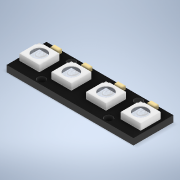
# Autodesk Inventor part: LED WS2812B
Saved by Autodesk Inventor 2020.1 (Build 241239000, 239)
## iProperties
Created: 2019-08-13
Part Number: LED WS2812B
Material: Generic
Document SubType Name: Modeling
Designer: Petar
Density: 1 g/cm^3
Appearance: Default
Author: Petar
Autodesk Inventor part; units mm, degrees
ref_plane "YZ Plane" through (0, 0, 0) normal (1, 0, 0) x (0, 1, 0)
ref_plane "XZ Plane" through (0, 0, 0) normal (0, 1, 0) x (-1, 0, 0)
sketch "Sketch1" plane through (0, 0, 0) normal (0, 1, 0) x (-1, 0, 0)
  line L0 (15.92, 5) -> (-15.92, 5)
  line L1 (-15.92, 5) -> (-15.92, -5)
  line L2 (-15.92, -5) -> (15.92, -5)
  line L3 (15.92, -5) -> (15.92, 5)
  line L4 (15.92, 5) -> (-15.92, -5) construction
  line L5 (-15.92, 5) -> (15.92, -5) construction
  line L6 (-10.87, -4.5) -> (-12.72, -4.5)
  line L7 (-12.72, -4.5) -> (-12.72, -3.5)
  line L8 (-12.72, -3.5) -> (-10.87, -3.5)
  line L9 (-10.87, -3.5) -> (-10.87, -4.5)
  circle A0 centre (-8.42, -3.75) radius 1
  line L10 (15.92, 0) -> (-15.92, 0) construction
  line L11 (0, -5) -> (0, 5) construction
  circle A1 centre (-8.42, 3.75) radius 1
  line L12 (-10.22, -2.5) -> (-15.22, -2.5)
  line L13 (-15.22, -2.5) -> (-15.22, 2.5)
  line L14 (-15.22, 2.5) -> (-10.22, 2.5)
  line L15 (-10.22, 2.5) -> (-10.22, -2.5)
  line L16 (-1.52, -2.5) -> (-6.52, -2.5)
  line L17 (-6.52, -2.5) -> (-6.52, 2.5)
  line L18 (-6.52, 2.5) -> (-1.52, 2.5)
  line L19 (-1.52, 2.5) -> (-1.52, -2.5)
  line L20 (7.18, -2.5) -> (2.18, -2.5)
  line L21 (2.18, -2.5) -> (2.18, 2.5)
  line L22 (2.18, 2.5) -> (7.18, 2.5)
  line L23 (7.18, 2.5) -> (7.18, -2.5)
  line L24 (15.22, -2.5) -> (10.22, -2.5)
  line L25 (10.22, -2.5) -> (10.22, 2.5)
  line L26 (10.22, 2.5) -> (15.22, 2.5)
  line L27 (15.22, 2.5) -> (15.22, -2.5)
  circle A2 centre (8.42, -3.75) radius 1
  circle A3 centre (8.42, 3.75) radius 1
  line L28 (-2.57, -4.5) -> (-4.42, -4.5)
  line L29 (-4.42, -4.5) -> (-4.42, -3.5)
  line L30 (-4.42, -3.5) -> (-2.57, -3.5)
  line L31 (-2.57, -3.5) -> (-2.57, -4.5)
  line L32 (5.73, -4.5) -> (3.88, -4.5)
  line L33 (3.88, -4.5) -> (3.88, -3.5)
  line L34 (3.88, -3.5) -> (5.73, -3.5)
  line L35 (5.73, -3.5) -> (5.73, -4.5)
  line L36 (13.42, -4.5) -> (11.57, -4.5)
  line L37 (11.57, -4.5) -> (11.57, -3.5)
  line L38 (11.57, -3.5) -> (13.42, -3.5)
  line L39 (13.42, -3.5) -> (13.42, -4.5)
  point P0 (0, 0)
  dimension "d0" = 31.84
  dimension "d1" = 10
  dimension "d2" = 1.85
  dimension "d3" = 1
  dimension "d4" = 7.5
  dimension "d5" = 7.5
  dimension "d6" = 2
  dimension "d7" = 3.2
  dimension "d8" = 0.5
  dimension "d9" = 5
  dimension "d10" = 0.7
  dimension "d11" = 3.7
  dimension "d12" = 0.7
  dimension "d14" = 6.45
  dimension "d15" = 6.45
  dimension "d16" = 2.5
  dimension "d18" = 3.7
  constraints: 80 end point, 18 parallel, 13 equal length, 9 horizontal, 9 perpendicular, 6 midpoint, 4 centre point, 3 symmetric about line, 2 collinear, 1 point on line, 7 other
  measures "d0" distance of L2.end L1.end
  measures "d1" distance of L1.end L0.end
  measures "d2" distance of L7.end L8.end
  measures "d3" distance of L6.end L7.end
  measures "d4" distance from line of L1 A0.centre
  measures "d5" distance of A1.centre A0.centre
  measures "d6" diameter of A0
  measures "d7" distance between parallel lines of L7 L1
  measures "d8" distance between parallel lines of L2 L6
  measures "d9" distance between parallel lines of L14 L12
  measures "d10" distance between parallel lines of L1 L13
  measures "d11" distance between parallel lines of L15 L17
  measures "d12" distance between parallel lines of L3 L27
  measures "d14" distance between parallel lines of L9 L29
  measures "d15" distance between parallel lines of L31 L33
  measures "d16" distance between parallel lines of L3 L39
  measures "d18" distance between parallel lines of L19 L21
extrude "Extrusion1" add sketch "Sketch1" against normal blind 1.6 contours L3 L2 L1 L0 | L6 L7 L8 L9 | L12 L13 L14 L15 | L16 L17 L18 L19 | L20 L21 L22 L23 | L24 L25 L26 L27 | L28 L29 L30 L31 | L32 L33 L34 L35 | L36 L37 L38 L39
extrude "Extrusion2" add sketch "Sketch1" along normal blind 1.6 contours L12 L13 L14 L15 | L16 L17 L18 L19 | L20 L21 L22 L23 | L24 L25 L26 L27
extrude "Extrusion3" add sketch "Sketch1" along normal blind 0.9 contours L6 L7 L8 L9 | L28 L29 L30 L31 | L32 L33 L34 L35 | L36 L37 L38 L39
sketch "Sketch2" plane through (0, 1.6, 0) normal (0, 1, 0) x (1, 0, 0)
  line L0 (-10.22, 2.5) -> (-15.22, 2.5) construction
  line L1 (-15.22, 2.5) -> (-15.22, -2.5) construction
  line L2 (-15.22, -2.5) -> (-10.22, -2.5) construction
  line L3 (-10.22, -2.5) -> (-10.22, 2.5) construction
  line L4 (-7.18, 2.5) -> (-7.18, -2.5) construction
  line L5 (-7.18, -2.5) -> (-2.18, -2.5) construction
  line L6 (-2.18, -2.5) -> (-2.18, 2.5) construction
  line L7 (-2.18, 2.5) -> (-7.18, 2.5) construction
  line L8 (6.52, 2.5) -> (1.52, 2.5) construction
  line L9 (1.52, 2.5) -> (1.52, -2.5) construction
  line L10 (1.52, -2.5) -> (6.52, -2.5) construction
  line L11 (6.52, -2.5) -> (6.52, 2.5) construction
  line L12 (10.22, 2.5) -> (10.22, -2.5) construction
  line L13 (10.22, -2.5) -> (15.22, -2.5) construction
  line L14 (15.22, -2.5) -> (15.22, 2.5) construction
  line L15 (15.22, 2.5) -> (10.22, 2.5) construction
  circle A0 centre (-12.72, 0) radius 1.75
  circle A1 centre (-4.68, 0) radius 1.75
  circle A2 centre (4.02, 0) radius 1.75
  circle A3 centre (12.72, 0) radius 1.75
  line L16 (-15.22, -2.5) -> (-15.22, 2.5) construction
  line L17 (-15.22, 1.5) -> (-14.22, 2.5)
  line L18 (-15.22, 2.5) -> (-10.22, 2.5) construction
  line L19 (-15.22, 2.5) -> (-15.22, 1.5)
  line L20 (-15.22, 2.5) -> (-14.22, 2.5)
  line L21 (-7.18, 2.5) -> (-7.18, 1.5)
  line L22 (-7.18, -2.5) -> (-7.18, 2.5) construction
  line L23 (-7.18, 2.5) -> (-2.18, 2.5) construction
  line L24 (-7.18, 2.5) -> (-6.18, 2.5)
  line L25 (-7.18, 1.5) -> (-6.18, 2.5)
  line L26 (1.52, 2.5) -> (1.52, 1.5)
  line L27 (1.52, 1.5) -> (2.52, 2.5)
  line L28 (1.52, -2.5) -> (1.52, 2.5) construction
  line L29 (2.52, 2.5) -> (1.52, 2.5)
  line L30 (10.22, 2.5) -> (10.22, 1.5)
  line L31 (10.22, -2.5) -> (10.22, 2.5) construction
  line L32 (10.22, 2.5) -> (15.22, 2.5) construction
  line L33 (10.22, 2.5) -> (11.22, 2.5)
  line L34 (10.22, 1.5) -> (11.22, 2.5)
  point P0 (0, 0)
  dimension "d25" = 3.5
  dimension "d26" = 45
  dimension "d27" = 1
  constraints: 24 end point, 8 point on line, 5 equal length, 4 centre point, 3 equal radius, 2 collinear, 1 horizontal, 1 parallel
  measures "d25" diameter of A0
  measures "d26" angle of L1 L17
  measures "d27" distance of L0.end L17.end
extrude "Extrusion4" cut sketch "Sketch2" against normal blind 0.2 contours L19 L20 L17 | L24 L25 L21 | L29 L27 L26 | L33 L34 L30
extrude "Extrusion5" cut sketch "Sketch2" against normal blind 0.8 contours A0 | A1 | A2 | A3
ref_plane "Work Plane1" through (0, 1.5, 0) normal (0, 1, 0) x (1, 0, 0)
sketch "Sketch3" plane through (0, 1.5, 0) normal (0, 1, 0) x (1, 0, 0)
  circle A0 centre (-12.72, 0) radius 1.75 projected
  circle A1 centre (-4.68, 0) radius 1.75 projected
  circle A2 centre (4.02, 0) radius 1.75 projected
  circle A3 centre (12.72, 0) radius 1.75 projected
  point P0 (0, 0)
extrude "Extrusion7" add sketch "Sketch3" against normal up to next
equation "\"d12\" = d10"
equation "\"d15\" = d14"
equation "\"d18\" = d11"
body "Solid1"
